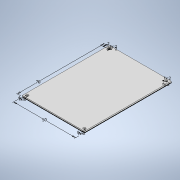
# Autodesk Inventor part: Enclosure Lid
Saved by Autodesk Inventor 2020.2 (Build 242310000, 310)
## iProperties
Created: 2020-09-23
Part Number: Enclosure Lid
Material: Generic
Document SubType Name: Modeling
Designer: johnf
Density: 1 g/cm^3
Appearance: Default
Author: johnf
Autodesk Inventor part; units mm, degrees
ref_plane "YZ Plane" through (0, 0, 0) normal (1, 0, 0) x (0, 1, 0)
ref_plane "XZ Plane" through (0, 0, 0) normal (0, 1, 0) x (-1, 0, 0)
ref_plane "XY Plane" through (0, 0, 0) normal (0, 0, 1) x (1, 0, 0)
sketch "Sketch1" plane through (0, 0, 0) normal (0, 1, 0) x (-1, 0, 0)
  line L0 (25, 35) -> (-25, 35)
  line L1 (-25, 35) -> (-25, -35)
  line L2 (-25, -35) -> (25, -35)
  line L3 (25, -35) -> (25, 35)
  line L4 (-25, 35) -> (25, -35) construction
  circle A0 centre (23, -33) radius 1
  circle A1 centre (-23, -33) radius 1
  circle A2 centre (-23, 33) radius 1
  circle A3 centre (23, 33) radius 1
  point P0 (0, 0)
  point P1 (0, 0)
  dimension "d0" = 70
  dimension "d1" = 50
  dimension "d17" = 2
  dimension "d18" = 2
  dimension "d21" = 2
  dimension "d22" = 2
  dimension "d23" = 2
  dimension "d25" = 2
  dimension "d26" = 2
  dimension "d27" = 2
  dimension "d28" = 2
  constraints: 10 end point, 4 centre point, 3 equal radius, 2 parallel, 1 coincident, 1 horizontal, 1 midpoint, 1 perpendicular
  measures "d0" distance of L2.end L0.start
  measures "d1" distance of L0.start L0.end
  measures "d17" distance from line of L2 A0.centre
  measures "d18" distance from line of A0.centre L3
  measures "d21" diameter of A0
  measures "d22" distance from line of A3.centre L0
  measures "d23" distance from line of L3 A3.centre
  measures "d25" distance from line of L0 A2.centre
  measures "d26" distance from line of L1 A2.centre
  measures "d27" distance from line of L1 A1.centre
  measures "d28" distance from line of L2 A1.centre
extrude "Extrusion1" add sketch "Sketch1" along normal blind 1
sketch "Sketch4" plane through (0, 0, 0) normal (0, -1, 0) x (1, 0, 0)
  line L0 (-19.8, 32.8) -> (19.8, 32.8)
  line L1 (22.8, 29.8) -> (22.8, -29.8)
  line L2 (19.8, -32.8) -> (-19.8, -32.8)
  line L3 (-22.8, -29.8) -> (-22.8, 29.8)
  line L4 (-22.8, 32.8) -> (22.8, -32.8) construction
  line L5 (-25, -35) -> (-25, 35) projected
  line L6 (-25, 35) -> (25, 35) projected
  arc A0 (-22.8, 29.8) -> (-19.8, 32.8) centre (-22.8, 32.8) ccw
  arc A1 (19.8, 32.8) -> (22.8, 29.8) centre (22.8, 32.8) ccw
  arc A2 (-19.8, -32.8) -> (-22.8, -29.8) centre (-22.8, -32.8) ccw
  arc A3 (22.8, -29.8) -> (19.8, -32.8) centre (22.8, -32.8) ccw
  line L7 (18.2174, 30.8) -> (-18.2174, 30.8)
  arc A4 (-20.8, 28.2174) -> (-18.2174, 30.8) centre (-22.8, 32.8) ccw
  line L8 (-20.8, 28.2174) -> (-20.8, -28.2174)
  arc A5 (-18.2174, -30.8) -> (-20.8, -28.2174) centre (-22.8, -32.8) ccw
  line L9 (-18.2174, -30.8) -> (18.2174, -30.8)
  arc A6 (20.8, -28.2174) -> (18.2174, -30.8) centre (22.8, -32.8) ccw
  line L10 (20.8, -28.2174) -> (20.8, 28.2174)
  arc A7 (18.2174, 30.8) -> (20.8, 28.2174) centre (22.8, 32.8) ccw
  point P0 (0, 0)
  point P1 (0, 0)
  dimension "d29" = 2.2
  dimension "d30" = 2.2
  dimension "d32" = 3
  dimension "d35" = 2
  constraints: 18 end point, 16 point on circle, 8 centre point, 8 point on line, 4 parallel, 3 coincident, 3 equal radius, 2 perpendicular, 1 horizontal, 1 midpoint, 7 other
  measures "d29" distance between parallel lines of L5 L3
  measures "d30" distance between parallel lines of L6 L0
  measures "d32" radius of A1
  measures "d35" distance between parallel lines of L0 L7
extrude "Extrusion4" add sketch "Sketch4" along normal blind 1
equation "\"d18\" = d17"
equation "\"d22\" = d17"
equation "\"d23\" = d17"
equation "\"d25\" = d17"
equation "\"d26\" = d17"
equation "\"d27\" = d17"
equation "\"d28\" = d17"
equation "\"d30\" = d29"
body "Solid1"
